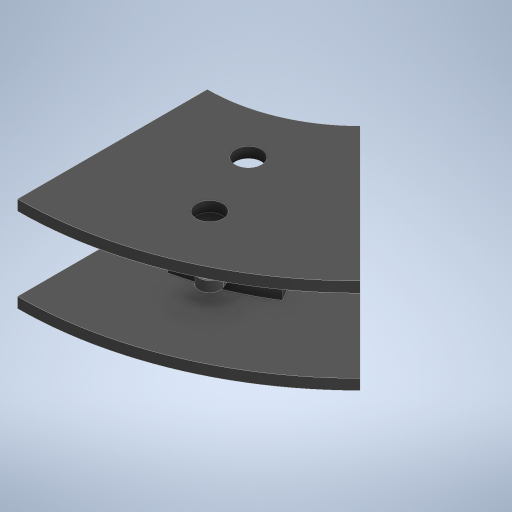
# Autodesk Inventor part: Roller Carousel Part
Saved by Autodesk Inventor 2023 (Build 270158000, 158)
## iProperties
Created: 2022-11-03
Part Number: Roller Carousel Part
Material: PLA Plastic
Document SubType Name: Modeling
Designer: cheng
Density: 0.373679 g/cm^3
Appearance: Generic
Mass: 326.783 g
Surface Area: 1739.53 cm^2
Volume: 874.504 cm^3
Author: cheng
Autodesk Inventor part; units mm, degrees
ref_plane "YZ Plane" through (0, 0, 0) normal (1, 0, 0) x (0, 1, 0)
ref_plane "XZ Plane" through (0, 0, 0) normal (0, 1, 0) x (-1, 0, 0)
ref_plane "XY Plane" through (0, 0, 0) normal (0, 0, 1) x (1, 0, 0)
sketch "Sketch1" plane through (0, 0, 0) normal (0, 1, 0) x (-1, 0, 0)
  circle A0 centre (0, 0) radius 325
  circle A1 centre (0, 0) radius 145
  line L0 (0, 0) -> (0, 325)
  line L1 (0, 0) -> (-325, 0)
  line L2 (0, 0) -> (-229.8097, 229.8097)
  line L3 (-124.3721, 300.2608) -> (-55.4891, 133.9625)
  circle A2 centre (-101.0284, 243.9042) radius 16 construction
  circle A3 centre (-75.006, 181.0804) radius 16 construction
  line L4 (-124.3721, 300.2608) -> (-55.4891, 133.9625)
  circle A4 centre (-101.0284, 243.9042) radius 16 construction
  circle A5 centre (-75.006, 181.0804) radius 16 construction
  circle A6 centre (-101.0284, 243.9042) radius 7.5
  circle A7 centre (-75.006, 181.0804) radius 10
  circle A8 centre (-101.0284, 243.9042) radius 10
  circle A9 centre (-75.006, 181.0804) radius 7.5
  circle A10 centre (-75.006, 181.0804) radius 10
  circle A11 centre (-101.0284, 243.9042) radius 10
  circle A12 centre (-101.0284, 243.9042) radius 7.5
  circle A13 centre (-75.006, 181.0804) radius 7.5
  line L5 (0, 145) -> (-102.5305, 102.5305)
  line L6 (-51.2652, 123.7652) -> (-73.3756, 177.1443)
  arc A14 (-89.9306, 217.1117) -> (-89.9306, 217.1117) centre (25.5588, -61.7044) ccw construction
  line L7 (-89.9306, 217.1117) -> (-100.6301, 242.9426)
  circle A15 centre (0, 0) radius 180
  circle A16 centre (0, 0) radius 280
  circle A17 centre (0, 0) radius 205
  circle A18 centre (0, 0) radius 255
  line L8 (-91.7896, 247.731) -> (-65.7672, 184.9072)
  line L9 (-110.2672, 240.0774) -> (-84.2447, 177.2536)
  line L10 (-91.7896, 247.731) -> (-65.7672, 184.9072)
  line L11 (-110.2672, 240.0774) -> (-84.2447, 177.2536)
  line L12 (-68.883, 166.2983) -> (-97.5843, 235.5893) construction
  line L13 (0, 0) -> (-70.3429, 317.2962)
  line L14 (0, 0) -> (-174.6224, 274.1022)
  point P0 (-108.3598, 242.3226)
  point P1 (-81.2257, 188.9108)
  point P2 (-93.7156, 245.5692)
  point P3 (-68.7834, 173.2522)
  point P4 (-102.2684, 253.827)
  point P5 (-66.5369, 175.763)
  point P6 (-99.7884, 233.9814)
  point P7 (-83.475, 186.3978)
  point P8 (-106.748, 231.5812)
  point P9 (-88.2704, 239.2349)
  point P10 (-69.1179, 192.9967)
  point P11 (-87.5955, 185.343)
  point P12 (-101.5282, 233.9167)
  point P13 (-93.6128, 237.1954)
  point P14 (-93.6128, 237.1954)
  point P15 (-74.3133, 191.0564)
  point P16 (-82.5498, 187.6447)
  point P17 (-74.3133, 191.0564)
  point P18 (-101.5282, 233.9167)
  point P19 (-82.5498, 187.6447)
  point P20 (-87.5955, 185.343)
  point P21 (-69.1179, 192.9967)
  point P22 (-88.2704, 239.2349)
  point P23 (-106.748, 231.5812)
  point P24 (-44.3701, 200.1407)
  point P25 (-55.1921, 248.9555)
  point P26 (-137.0114, 215.0648)
  point P27 (-110.1464, 172.8952)
  dimension "d0" = 650
  dimension "d1" = 180
  dimension "d2" = 45
  dimension "d4" = 32
  dimension "d5" = 32
  dimension "d7" = 32
  dimension "d8" = 32
  dimension "d11" = 15
  dimension "d12" = 20
  dimension "d14" = 15
  dimension "d15" = 20
  dimension "d16" = 20
  dimension "d17" = 20
  dimension "d18" = 15
  dimension "d19" = 15
  dimension "d38" = 0
  dimension "d101" = 25
  dimension "d102" = 25
  dimension "d112" = 100
  dimension "d129" = 35
  dimension "d146" = 20
  constraints: 30 end point, 23 point on circle, 16 centre point, 14 coincident, 10 tangent, 8 point on line, 3 midpoint, 2 perpendicular, 1 collinear, 1 line through centre, 1 vertical, 21 other
  measures "d2" angle of L2 L0
  measures "d4" diameter of A2
  measures "d5" diameter of A3
  measures "d7" diameter of A4
  measures "d8" diameter of A5
  measures "d11" diameter of A6
  measures "d12" diameter of A7
  measures "d14" diameter of A9
  measures "d15" diameter of A8
  measures "d16" diameter of A10
  measures "d17" diameter of A11
  measures "d18" diameter of A13
  measures "d19" diameter of A12
  measures "d38" distance between parallel lines of L3 L4
  measures "d146" angle of L14 L13
extrude "Extrusion1" add sketch "Sketch1" along normal blind 30 contours L13 A17 L8 A18 | A8 A18 L3 A6 | L3 A6 A18 A8 | L8 A17 A7 L3 A8 A18 | A18 A8 L8 | A18 L9 A17 L14 | A8 A18 L9 | A8 L3 A18 | L8 A7 A17 | A18 A8 L3 A7 A17 L9 | A18 L3 A8 | A17 L3 A7 | A7 L3 A9 A17 | A17 A7 L9 | L3 A17 A7 | L3 A9 A7 A17
sketch "Sketch5" plane through (0, 30, 0) normal (0, 1, 0) x (1, 0, 0)
  line L0 (87.5955, -185.343) -> (84.2447, -177.2536) projected
  arc A0 (84.2447, -177.2536) -> (65.7672, -184.9072) centre (75.006, -181.0804) ccw projected
  line L1 (65.7672, -184.9072) -> (69.1179, -192.9967) projected
  arc A1 (44.3701, -200.1407) -> (69.1179, -192.9967) centre (0, 0) ccw projected
  line L2 (44.3701, -200.1407) -> (55.1921, -248.9555) projected
  arc A2 (55.1921, -248.9555) -> (88.2704, -239.2349) centre (0, 0) ccw projected
  line L3 (88.2704, -239.2349) -> (91.7896, -247.731) projected
  arc A3 (91.7896, -247.731) -> (110.2672, -240.0774) centre (101.0284, -243.9042) ccw projected
  line L4 (110.2672, -240.0774) -> (106.748, -231.5812) projected
  arc A4 (106.748, -231.5812) -> (137.0114, -215.0648) centre (0, 0) ccw projected
  line L5 (137.0114, -215.0648) -> (110.1464, -172.8952) projected
  arc A5 (87.5955, -185.343) -> (110.1464, -172.8952) centre (0, 0) ccw projected
  circle A6 centre (101.0284, -243.9042) radius 7.5 projected
  circle A7 centre (75.006, -181.0804) radius 7.5 projected
  circle A8 centre (0, 0) radius 205
  circle A9 centre (0, 0) radius 255
  line L6 (0, 0) -> (55.1921, -248.9555)
  line L7 (0, 0) -> (137.0114, -215.0648)
  point P0 (55.1921, -248.9555)
  point P1 (137.0114, -215.0648)
  dimension "d147" = 410
  dimension "d148" = 510
  constraints: 4 end point, 2 centre point, 2 coincident, 1 collinear
  measures "d147" diameter of A8
  measures "d148" diameter of A9
extrude "Top Pillar" add sketch "Sketch5" along normal blind 20 contours A5 L5 A4 A9 A2 L2 A1 A8
sketch "Sketch6" plane through (0, 0, 0) normal (0, -1, 0) x (1, 0, 0)
  line L0 (87.5955, 185.343) -> (84.2447, 177.2536) projected
  arc A0 (110.1464, 172.8952) -> (87.5955, 185.343) centre (0, 0) ccw projected
  line L1 (137.0114, 215.0648) -> (110.1464, 172.8952) projected
  arc A1 (137.0114, 215.0648) -> (106.748, 231.5812) centre (0, 0) ccw projected
  line L2 (110.2672, 240.0774) -> (106.748, 231.5812) projected
  arc A2 (110.2672, 240.0774) -> (91.7896, 247.731) centre (101.0284, 243.9042) ccw projected
  line L3 (88.2704, 239.2349) -> (91.7896, 247.731) projected
  arc A3 (88.2704, 239.2349) -> (55.1921, 248.9555) centre (0, 0) ccw projected
  line L4 (44.3701, 200.1407) -> (55.1921, 248.9555) projected
  arc A4 (69.1179, 192.9967) -> (44.3701, 200.1407) centre (0, 0) ccw projected
  line L5 (65.7672, 184.9072) -> (69.1179, 192.9967) projected
  arc A5 (65.7672, 184.9072) -> (84.2447, 177.2536) centre (75.006, 181.0804) ccw projected
  circle A6 centre (101.0284, 243.9042) radius 7.5 projected
  circle A7 centre (75.006, 181.0804) radius 7.5 projected
  circle A8 centre (0, 0) radius 205
  circle A9 centre (0, 0) radius 255
  line L6 (44.3701, 200.1407) -> (55.1921, 248.9555) projected
  line L7 (0, 0) -> (55.1921, 248.9555)
  line L8 (0, 0) -> (137.0114, 215.0648)
  point P0 (106.748, 231.5812)
  point P1 (69.1179, 192.9967)
  dimension "d149" = 510
  dimension "d150" = 410
  constraints: 4 end point, 2 centre point, 2 coincident, 1 collinear
  measures "d149" diameter of A9
  measures "d150" diameter of A8
extrude "Lower Pillar" add sketch "Sketch6" along normal blind 20 contours A8 A4 L4 A3 A9 A1 L1 A0
sketch "Sketch7" plane through (0, 50, 0) normal (0, 1, 0) x (1, 0, 0)
  circle A0 centre (0, 0) radius 145
  circle A1 centre (0, 0) radius 325
  arc A2 (84.2447, -177.2536) -> (65.7672, -184.9072) centre (75.006, -181.0804) ccw construction
  circle A3 centre (101.0284, -243.9042) radius 7.5 construction
  arc A4 (84.2447, -177.2536) -> (65.7672, -184.9072) centre (75.006, -181.0804) ccw construction
  line L0 (0, 0) -> (325, 0) construction
  circle A5 centre (75.006, -181.0804) radius 7.5 projected
  circle A6 centre (101.0284, -243.9042) radius 7.5 projected
  circle A7 centre (101.0284, -243.9042) radius 12.5
  circle A8 centre (75.006, -181.0804) radius 7.5 projected
  circle A9 centre (75.006, -181.0804) radius 12.5
  line L1 (137.0114, -215.0648) -> (110.1464, -172.8952) projected
  arc A10 (44.3701, -200.1407) -> (110.1464, -172.8952) centre (0, 0) ccw projected
  line L2 (44.3701, -200.1407) -> (55.1921, -248.9555) projected
  arc A11 (55.1921, -248.9555) -> (137.0114, -215.0648) centre (0, 0) ccw projected
  circle A12 centre (0, 0) radius 230
  line L3 (0, 0) -> (124.3721, -300.2608) construction
  line L4 (0, 0) -> (0, -325)
  line L5 (0, 0) -> (229.8097, -229.8097)
  point P0 (229.8097, -229.8097)
  point P1 (102.5305, -102.5305)
  point P2 (0, -145)
  dimension "d105" = 650
  dimension "d107" = 180
  dimension "d115" = 5
  dimension "d116" = 5
  dimension "d151" = 460
  dimension "d153" = 45
  constraints: 8 end point, 5 centre point, 5 coincident, 5 point on circle, 1 horizontal, 1 point on line, 1 vertical
  measures "d105" diameter of A1
  measures "d107" radial gap between concentric circles of A0 A1
  measures "d115" radial gap between concentric circles of A9 A5
  measures "d116" radial gap between concentric circles of A7 A3
  measures "d151" diameter of A12
  measures "d153" angle of L4 L5
extrude "Top Face" add sketch "Sketch7" along normal blind 10 contours A0 L5 A12 L1 A10 A9 L2 L4 | A12 L2 A11 A7 L1 L5 A1 L4 | A12 L1 A11 A7 L2 | L2 A10 A9 L1 A12
sketch "Sketch9" plane through (0, -20, 0) normal (0, -1, 0) x (1, 0, 0)
  arc A0 (229.8097, 229.8097) -> (0, 325) centre (0, 0) ccw projected
  line L0 (229.8097, 229.8097) -> (102.5305, 102.5305) projected
  arc A1 (102.5305, 102.5305) -> (0, 145) centre (0, 0) ccw projected
  line L1 (0, 145) -> (0, 325) projected
extrude "Extrusion5" add sketch "Sketch9" along normal blind 10
sketch "Sketch11" plane through (82.4407, 0, 172.8982) normal (0.9238795, 0, -0.3826834) x (-0.3826834, 0, -0.9238795)
  line L0 (5.2858, 0) -> (5.2858, 30) projected
  line L1 (5.2858, 0) -> (5.2858, 30) projected
  line L2 (5.2858, 0) -> (5.2858, 30) projected
  line L3 (-82.7142, 0) -> (-82.7142, 30) projected
  line L4 (5.2858, 30) -> (-4.7142, 30) projected
  line L5 (-82.7142, 30) -> (5.2858, 30)
  line L6 (5.2858, 0) -> (-4.7142, 0) projected
  line L7 (-82.7142, 0) -> (5.2858, 0)
  line L8 (-82.7142, 0) -> (-82.7142, 30) projected
  line L9 (-82.7142, 15) -> (5.2858, 15) construction
  line L10 (5.2858, 0) -> (5.2858, 30) projected
  line L11 (-82.7142, 0) -> (-82.7142, 30) projected
  line L12 (-82.7142, 20) -> (5.2858, 20)
  line L13 (5.2858, 0) -> (5.2858, 30) projected
  line L14 (-82.7142, 0) -> (-82.7142, 30) projected
  line L15 (-82.7142, 10) -> (5.2858, 10)
  line L16 (-38.7142, 15) -> (-38.7142, 50) construction
  line L17 (-108.975, 50) -> (57.3233, 50) projected
  line L18 (-38.7142, 15) -> (-38.7142, -26.3002) construction
  line L19 (-63.518, 0) -> (-63.518, 30) projected
  line L20 (-63.518, 30) -> (-63.518, 0)
  line L21 (-13.4701, 0) -> (-13.4701, 30) projected
  line L22 (-13.4701, 30) -> (-13.4701, 0)
  line L23 (-63.518, 30) -> (-63.7142, 50)
  line L24 (-63.7142, -20) -> (-63.7142, 50) projected
  line L25 (-13.4701, 30) -> (-13.7142, 50)
  line L26 (-13.7142, 50) -> (-13.7142, -20) projected
  line L27 (-13.4701, 0) -> (-4.7142, 0) projected
  line L28 (-13.4701, 0) -> (-13.7142, -20)
  line L29 (-63.7142, -20) -> (-63.7142, 50) projected
  line L30 (-63.518, 0) -> (-63.7142, -20)
  line L31 (-63.7142, -20) -> (-63.7142, 50) projected
  line L32 (-63.7142, -20) -> (-59.8401, -20) projected
  line L33 (-63.7142, -20) -> (-13.7142, -20)
  line L34 (-28.7142, 50) -> (-28.7142, -20)
  line L35 (-48.7142, 50) -> (-48.7142, -20)
  line L36 (-13.5222, 50) -> (7.7858, 50) projected
  line L37 (-13.4701, 30) -> (-4.7142, 30) projected
  line L38 (-9.0921, 0) -> (-9.0921, -20)
  line L39 (-9.3362, 50) -> (-9.0921, 30)
  line L40 (5.2858, 30) -> (10.2858, 30)
  line L41 (10.2858, 30) -> (10.2858, 0)
  line L42 (5.2858, 10) -> (10.2858, 10)
  line L43 (5.2858, 20) -> (10.2858, 20)
  line L44 (-10.5998, -20) -> (-13.7142, -20) projected
  line L45 (-9.0921, -20) -> (-13.7142, -20)
  point P0 (-38.7142, 32.5)
  point P1 (-13.4701, 20)
  point P2 (-13.4701, 10)
  point P3 (5.2858, 10)
  point P4 (5.2858, 20)
  point P5 (-28.7142, 20)
  point P6 (-28.7142, 10)
  point P7 (-13.7142, 10)
  point P8 (-13.7142, 20)
  point P9 (-28.7142, 0)
  point P10 (-13.7142, 0)
  point P11 (-48.7142, 0)
  point P12 (-59.8401, -20)
  point P13 (-28.7142, 30)
  point P14 (-13.7142, 30)
  point P15 (-48.7142, 30)
  point P16 (-48.7142, 10)
  point P17 (-48.7142, 20)
  point P18 (-63.518, 20)
  point P19 (-63.518, 10)
  point P20 (-63.7142, 10)
  point P21 (-63.7142, 20)
  point P22 (5.2858, 20)
  point P23 (5.2858, 10)
  point P24 (-9.0921, 30)
  point P25 (-9.3362, 50)
  point P26 (-9.0921, 0)
  dimension "d159" = 5
  dimension "d160" = 5
  dimension "d162" = 10
  dimension "d163" = 10
  dimension "d164" = 4.3777
  dimension "d165" = 0.699
  dimension "d166" = 5
  constraints: 46 end point, 9 point on line, 5 midpoint, 4 horizontal, 4 perpendicular, 3 vertical, 2 collinear, 1 parallel, 14 other
  measures "d159" distance between parallel lines of L9 L12
  measures "d160" distance between parallel lines of L9 L15
  measures "d162" distance from line of point (-38.714, 32.5) L34
  measures "d163" distance between parallel lines of L16 L35
  measures "d164" distance between parallel lines of L39 L25
  measures "d165" angle of L38 L28
sketch3d "3D Sketch3"
  arc A0 (102.5305, 50, 102.5305) -> (0, 50, 145) centre (0, 50, 0) ccw
sweep "Sweep3" cut profiles "Sketch11" path "3D Sketch3" contours L15 L21 L12 L0 | L0 L43 L41 L42 | L15 L26 L12 L21 | L38 L45 L44 L28 L7 | L15 L34 L12 L26 | L28 L26 L7 | L25 L17 L39 L5 | L5 L26 L25 | L26 L33 L34 L7 | L5 L34 L17 L26 | L15 L19 L12 L35 | L15 L24 L12 L19 | L35 L33 L32 L30 L7 | L5 L23 L17 L35 | L15 L3 L12 L24
sketch "Sketch17" plane through (87.5955, 10, 185.343) normal (0, 1, 0) x (0.9238795, 0, -0.3826834)
  line L0 (25.5979, 2.8704) -> (28.242, -12.1255) projected
  arc A0 (0, 0) -> (25.5979, 2.8704) centre (-10, 204.756) ccw projected
  line L1 (0, 8.756) -> (0, 0) projected
  arc A1 (0, 8.756) -> (-20, 8.756) centre (-10, 8.756) ccw projected
  line L2 (-20, 0) -> (-20, 8.756) projected
  arc A2 (-45.5979, 2.8704) -> (-20, 0) centre (-10, 204.756) ccw projected
  line L3 (-48.242, -12.1255) -> (-45.5979, 2.8704) projected
  arc A3 (-48.242, -12.1255) -> (28.242, -12.1255) centre (-10, 204.756) ccw projected
  circle A4 centre (-10, 8.756) radius 7.5 projected
  line L4 (-54.2803, -46.37) -> (-51.7117, -31.803) projected
  arc A5 (-54.2803, -46.37) -> (-20, -50.0479) centre (-10, 204.756) ccw projected
  line L5 (-20, -59.244) -> (-20, -50.0479) projected
  arc A6 (-20, -59.244) -> (0, -59.244) centre (-10, -59.244) ccw projected
  line L6 (0, -50.0479) -> (0, -59.244) projected
  arc A7 (0, -50.0479) -> (34.2803, -46.37) centre (-10, 204.756) ccw projected
  line L7 (31.7117, -31.803) -> (34.2803, -46.37) projected
  arc A8 (-51.7117, -31.803) -> (31.7117, -31.803) centre (-10, 204.756) ccw projected
  circle A9 centre (-10, -59.244) radius 7.5 projected
  arc A10 (-45.5979, 2.8704) -> (-20, 0) centre (-10, 204.756) ccw projected
  line L8 (-20, 8.756) -> (-20, 0) projected
  arc A11 (0, -50.0479) -> (34.2803, -46.37) centre (-10, 204.756) ccw projected
  line L9 (-20, -50.0479) -> (-20, -59.244) projected
  line L10 (0, 0) -> (0, -50.0479)
  line L11 (-20, 0) -> (-20, -50.0479)
  point P0 (0, -35.244)
  point P1 (-20, -35.244)
  point P2 (0, -15.244)
  point P3 (-20, -15.244)
  constraints: 4 end point, 1 parallel, 1 vertical
extrude "Extrusion11" cut sketch "Sketch17" along normal mid plane 40 contours L0 A3 L10 A0 | A3 L3 A2 L11 | A8 L7 A7 L10 | L11 A5 L4 A8
sketch "Sketch18" plane through (93.4292, 10, 199.4267) normal (0, 1, 0) x (0.9238795, 0, -0.3826834)
  circle A0 centre (-10, 24) radius 7.5 projected
  circle A1 centre (-10, 24) radius 7.5
  circle A2 centre (-10, 24) radius 8.5
  circle A3 centre (-10, -44) radius 7.5 projected
  circle A4 centre (-10, -44) radius 7.5
  circle A5 centre (-10, -44) radius 8.5
  point P0 (-10, 220)
  dimension "d169" = 15
  dimension "d170" = 15
  dimension "d171" = 1
  dimension "d172" = 1
  constraints: 4 centre point, 4 coincident
  measures "d169" diameter of A0
  measures "d170" diameter of A3
  measures "d171" radial gap between concentric circles of A3 A5
  measures "d172" radial gap between concentric circles of A2 A0
extrude "Extrusion12" add sketch "Sketch18" along normal blind 0.5 and the other way blind 10.5
sketch "Sketch19" plane through (0, 30, 0) normal (0, 1, 0) x (1, 0, 0)
  circle A0 centre (75.006, -181.0804) radius 7.5 projected
  circle A1 centre (75.006, -181.0804) radius 7.5
  circle A2 centre (101.0284, -243.9042) radius 7.5 projected
  circle A3 centre (101.0284, -243.9042) radius 7.5
  circle A4 centre (101.0284, -243.9042) radius 7.5
  circle A5 centre (101.0284, -243.9042) radius 8.5
  circle A6 centre (75.006, -181.0804) radius 8.5
  point P0 (0, 0)
  dimension "d177" = 1
  dimension "d178" = 1
  constraints: 5 centre point, 5 coincident, 1 concentric
  measures "d177" radial gap between concentric circles of A0 A6
  measures "d178" radial gap between concentric circles of A5 A2
extrude "Extrusion13" add sketch "Sketch19" along normal blind 0.5 and the other way blind 10.5
sketch "Sketch20" plane through (0, -20, 0) normal (0, 1, 0) x (1, 0, 0)
  circle A0 centre (0, 0) radius 145
  circle A1 centre (0, 0) radius 325
  arc A2 (0, -325) -> (229.8097, -229.8097) centre (0, 0) ccw projected
  line L0 (0, 0) -> (0, -325) construction
  line L1 (102.5305, -102.5305) -> (229.8097, -229.8097) projected
  line L2 (0, 0) -> (229.8097, -229.8097) construction
  line L3 (0, 0) -> (124.3721, -300.2608) construction
  line L4 (127.5467, -127.5467) -> (0, -180.3783) construction
  line L5 (228.0336, -228.0336) -> (0, -322.4881) construction
  point P0 (55.4891, -133.9625)
  point P1 (63.7734, -153.9625)
  point P2 (114.0168, -275.2608)
  dimension "d183" = 290
  dimension "d184" = 650
  dimension "d189" = 20
  dimension "d190" = 25
  constraints: 10 end point, 7 point on line, 3 coincident, 2 centre point, 2 midpoint, 2 perpendicular, 2 point on circle, 1 collinear, 1 vertical
  measures "d183" diameter of A0
  measures "d184" diameter of A1
  measures "d189" vertical distance of point (63.773, -153.963) A0.end
  measures "d190" vertical distance of point (124.372, -300.261) point (114.017, -275.261)
sketch "Sketch21" plane through (0, 50, 0) normal (0, -1, 0) x (1, 0, 0)
  line L0 (127.5467, 127.5467) -> (0, 180.3783) construction
  line L1 (228.0336, 228.0336) -> (0, 322.4881) construction
  line L2 (0, 0) -> (124.3721, 300.2608) construction
body "Solid1"
